Autodesk Inventor part; units mm, degrees
(part 2 of 3)
  line L983 (33.9182, 21.8053) -> (33.8229, 21.957)
  line L984 (33.8229, 21.957) -> (33.7637, 22.1261)
  line L985 (33.7637, 22.1261) -> (33.7437, 22.3041)
  line L986 (33.7437, 22.3041) -> (33.7637, 22.4821)
  line L987 (33.7637, 22.4821) -> (33.8229, 22.6512)
  line L988 (33.8229, 22.6512) -> (33.9182, 22.8029)
  line L989 (33.9182, 22.8029) -> (34.0449, 22.9296)
  line L990 (34.0449, 22.9296) -> (34.1966, 23.0249)
  line L991 (34.1966, 23.0249) -> (34.3656, 23.084)
  line L992 (34.3656, 23.084) -> (34.5437, 23.1041)
  line L993 (34.5437, 23.1041) -> (34.7217, 23.084)
  line L994 (57.188, 32.7799) -> (57.3571, 32.7208)
  line L995 (57.3571, 32.7208) -> (57.5088, 32.6255)
  line L996 (57.5088, 32.6255) -> (57.6355, 32.4988)
  line L997 (57.6355, 32.4988) -> (57.7308, 32.3471)
  line L998 (57.7308, 32.3471) -> (57.7899, 32.178)
  line L999 (57.7899, 32.178) -> (57.81, 32)
  line L1000 (57.81, 32) -> (57.7899, 31.822)
  line L1001 (57.7899, 31.822) -> (57.7308, 31.6529)
  line L1002 (57.7308, 31.6529) -> (57.6355, 31.5012)
  line L1003 (57.6355, 31.5012) -> (57.51, 31.3757)
  line L1004 (57.51, 31.3757) -> (57.51, 30.7979)
  line L1005 (57.51, 30.7979) -> (57.5024, 30.745)
  line L1006 (57.5024, 30.745) -> (57.4986, 30.6916)
  line L1007 (57.4986, 30.6916) -> (57.4923, 30.6748)
  line L1008 (57.4923, 30.6748) -> (57.4897, 30.6571)
  line L1009 (57.4897, 30.6571) -> (57.4675, 30.6084)
  line L1010 (57.4675, 30.6084) -> (57.4488, 30.5583)
  line L1011 (57.4488, 30.5583) -> (57.4381, 30.5439)
  line L1012 (57.4381, 30.5439) -> (57.4306, 30.5276)
  line L1013 (57.4306, 30.5276) -> (57.3956, 30.4872)
  line L1014 (57.3956, 30.4872) -> (57.3636, 30.4444)
  line L1015 (57.3636, 30.4444) -> (52.3656, 25.4464)
  line L1016 (52.3656, 25.4464) -> (52.3228, 25.4144)
  line L1017 (52.3228, 25.4144) -> (52.2824, 25.3794)
  line L1018 (52.2824, 25.3794) -> (52.2661, 25.3719)
  line L1019 (52.2661, 25.3719) -> (52.2517, 25.3612)
  line L1020 (52.2517, 25.3612) -> (52.2016, 25.3425)
  line L1021 (52.2016, 25.3425) -> (52.1529, 25.3203)
  line L1022 (52.1529, 25.3203) -> (52.1352, 25.3177)
  line L1023 (52.1352, 25.3177) -> (52.1184, 25.3114)
  line L1024 (52.1184, 25.3114) -> (52.065, 25.3076)
  line L1025 (52.065, 25.3076) -> (52.0121, 25.3)
  line L1026 (52.0121, 25.3) -> (32.5037, 25.3)
  line L1027 (32.5037, 25.3) -> (32.5037, 22.9283)
  line L1028 (32.5037, 22.9283) -> (32.6291, 22.8029)
  line L1029 (32.6291, 22.8029) -> (32.7244, 22.6512)
  line L1030 (32.7244, 22.6512) -> (32.7836, 22.4821)
  line L1031 (32.7836, 22.4821) -> (32.8037, 22.3041)
  line L1032 (32.8037, 22.3041) -> (32.7836, 22.1261)
  line L1033 (32.7836, 22.1261) -> (32.7244, 21.957)
  line L1034 (32.7244, 21.957) -> (32.6291, 21.8053)
  line L1035 (32.6291, 21.8053) -> (32.5025, 21.6786)
  line L1036 (32.5025, 21.6786) -> (32.3508, 21.5833)
  line L1037 (32.3508, 21.5833) -> (32.1817, 21.5241)
  line L1038 (32.1817, 21.5241) -> (32.0037, 21.5041)
  line L1039 (32.0037, 21.5041) -> (31.8256, 21.5241)
  line L1040 (31.8256, 21.5241) -> (31.6566, 21.5833)
  line L1041 (31.6566, 21.5833) -> (31.5049, 21.6786)
  line L1042 (31.5049, 21.6786) -> (31.3782, 21.8053)
  line L1043 (31.3782, 21.8053) -> (31.2829, 21.957)
  line L1044 (31.2829, 21.957) -> (31.2237, 22.1261)
  line L1045 (31.2237, 22.1261) -> (31.2037, 22.3041)
  line L1046 (31.2037, 22.3041) -> (31.2237, 22.4821)
  line L1047 (31.2237, 22.4821) -> (31.2829, 22.6512)
  line L1048 (31.2829, 22.6512) -> (31.3782, 22.8029)
  line L1049 (31.3782, 22.8029) -> (31.5037, 22.9283)
  line L1050 (31.5037, 22.9283) -> (31.5037, 25.3601)
  line L1051 (31.5037, 25.3601) -> (29.8918, 25.3601)
  line L1052 (29.8918, 25.3601) -> (29.8621, 25.3045)
  line L1053 (29.8621, 25.3045) -> (29.7377, 25.153)
  line L1054 (29.7377, 25.153) -> (29.5862, 25.0286)
  line L1055 (29.5862, 25.0286) -> (29.4133, 24.9362)
  line L1056 (29.4133, 24.9362) -> (29.2257, 24.8793)
  line L1057 (29.2257, 24.8793) -> (29.0306, 24.8601)
  line L1058 (29.0306, 24.8601) -> (28.8355, 24.8793)
  line L1059 (28.8355, 24.8793) -> (28.6479, 24.9362)
  line L1060 (28.6479, 24.9362) -> (28.475, 25.0286)
  line L1061 (28.475, 25.0286) -> (28.3235, 25.153)
  line L1062 (28.3235, 25.153) -> (28.1991, 25.3045)
  line L1063 (28.1991, 25.3045) -> (28.1694, 25.3601)
  line L1064 (28.1694, 25.3601) -> (27.5999, 25.3601)
  line L1065 (27.5999, 25.3601) -> (27.547, 25.3677)
  line L1066 (27.547, 25.3677) -> (27.4936, 25.3715)
  line L1067 (27.4936, 25.3715) -> (27.4768, 25.3778)
  line L1068 (27.4768, 25.3778) -> (27.459, 25.3803)
  line L1069 (27.459, 25.3803) -> (27.4104, 25.4026)
  line L1070 (27.4104, 25.4026) -> (27.3603, 25.4213)
  line L1071 (27.3603, 25.4213) -> (27.3459, 25.432)
  line L1072 (27.3459, 25.432) -> (27.3296, 25.4395)
  line L1073 (27.3296, 25.4395) -> (27.2892, 25.4745)
  line L1074 (27.2892, 25.4745) -> (27.2464, 25.5065)
  line L1075 (27.2464, 25.5065) -> (21.5935, 31.1594)
  line L1076 (21.5935, 31.1594) -> (21.51, 31.15)
  line L1077 (21.51, 31.15) -> (21.332, 31.1701)
  line L1078 (21.332, 31.1701) -> (21.1629, 31.2292)
  line L1079 (21.1629, 31.2292) -> (21.0112, 31.3245)
  line L1080 (21.0112, 31.3245) -> (20.8857, 31.45)
  line L1081 (20.8857, 31.45) -> (20.7171, 31.45)
  line L1082 (20.7171, 31.45) -> (15.5506, 26.2835)
  line L1083 (15.5506, 26.2835) -> (15.56, 26.2)
  line L1084 (15.56, 26.2) -> (15.5399, 26.022)
  line L1085 (15.5399, 26.022) -> (15.4808, 25.8529)
  line L1086 (15.4808, 25.8529) -> (15.3855, 25.7012)
  line L1087 (15.3855, 25.7012) -> (15.2588, 25.5745)
  line L1088 (15.2588, 25.5745) -> (15.1071, 25.4792)
  line L1089 (15.1071, 25.4792) -> (14.938, 25.4201)
  line L1090 (14.938, 25.4201) -> (14.76, 25.4)
  line L1091 (14.76, 25.4) -> (14.582, 25.4201)
  line L1092 (14.582, 25.4201) -> (14.4129, 25.4792)
  line L1093 (14.4129, 25.4792) -> (14.2612, 25.5745)
  line L1094 (14.2612, 25.5745) -> (14.1345, 25.7012)
  line L1095 (14.1345, 25.7012) -> (14.0392, 25.8529)
  line L1096 (14.0392, 25.8529) -> (13.9801, 26.022)
  line L1097 (13.9801, 26.022) -> (13.96, 26.2)
  line L1098 (13.96, 26.2) -> (13.9801, 26.378)
  line L1099 (13.9801, 26.378) -> (14.0392, 26.5471)
  line L1100 (14.0392, 26.5471) -> (14.1345, 26.6988)
  line L1101 (14.1345, 26.6988) -> (14.2612, 26.8255)
  line L1102 (14.2612, 26.8255) -> (14.4129, 26.9208)
  line L1103 (14.4129, 26.9208) -> (14.582, 26.9799)
  line L1104 (14.582, 26.9799) -> (14.76, 27)
  line L1105 (14.76, 27) -> (14.8435, 26.9906)
  line L1106 (14.8435, 26.9906) -> (20.1564, 32.3036)
  line L1107 (20.1564, 32.3036) -> (20.1993, 32.3356)
  line L1108 (20.1993, 32.3356) -> (20.2397, 32.3706)
  line L1109 (20.2397, 32.3706) -> (20.256, 32.3781)
  line L1110 (20.256, 32.3781) -> (20.2704, 32.3888)
  line L1111 (20.2704, 32.3888) -> (20.3205, 32.4075)
  line L1112 (20.3205, 32.4075) -> (20.3691, 32.4297)
  line L1113 (20.3691, 32.4297) -> (20.3869, 32.4323)
  line L1114 (20.3869, 32.4323) -> (20.4037, 32.4386)
  line L1115 (20.4037, 32.4386) -> (20.4571, 32.4424)
  line L1116 (20.4571, 32.4424) -> (20.51, 32.45)
  line L1117 (20.51, 32.45) -> (20.8857, 32.45)
  line L1118 (20.8857, 32.45) -> (21.0112, 32.5755)
  line L1119 (21.0112, 32.5755) -> (21.1629, 32.6708)
  line L1120 (21.1629, 32.6708) -> (21.332, 32.7299)
  line L1121 (21.332, 32.7299) -> (21.51, 32.75)
  line L1122 (21.51, 32.75) -> (21.688, 32.7299)
  line L1123 (21.688, 32.7299) -> (21.8571, 32.6708)
  line L1124 (21.8571, 32.6708) -> (22.0088, 32.5755)
  line L1125 (22.0088, 32.5755) -> (22.1355, 32.4488)
  line L1126 (22.1355, 32.4488) -> (22.2308, 32.2971)
  line L1127 (22.2308, 32.2971) -> (22.2899, 32.128)
  line L1128 (22.2899, 32.128) -> (22.31, 31.95)
  line L1129 (22.31, 31.95) -> (22.3006, 31.8665)
  line L1130 (22.3006, 31.8665) -> (27.807, 26.3601)
  line L1131 (27.807, 26.3601) -> (28.1694, 26.3601)
  line L1132 (28.1694, 26.3601) -> (28.1991, 26.4157)
  line L1133 (28.1991, 26.4157) -> (28.3235, 26.5672)
  line L1134 (28.3235, 26.5672) -> (28.475, 26.6916)
  line L1135 (28.475, 26.6916) -> (28.6479, 26.784)
  line L1136 (28.6479, 26.784) -> (28.8355, 26.8409)
  line L1137 (28.8355, 26.8409) -> (29.0306, 26.8601)
  line L1138 (29.0306, 26.8601) -> (29.2257, 26.8409)
  line L1139 (29.2257, 26.8409) -> (29.4133, 26.784)
  line L1140 (29.4133, 26.784) -> (29.5862, 26.6916)
  line L1141 (29.5862, 26.6916) -> (29.7377, 26.5672)
  line L1142 (29.7377, 26.5672) -> (29.8621, 26.4157)
  line L1143 (29.8621, 26.4157) -> (29.8918, 26.3601)
  line L1144 (29.8918, 26.3601) -> (31.8972, 26.3601)
  line L1145 (31.8972, 26.3601) -> (31.9502, 26.3525)
  line L1146 (31.9502, 26.3525) -> (32.0035, 26.3487)
  line L1147 (32.0035, 26.3487) -> (32.0203, 26.3424)
  line L1148 (32.0203, 26.3424) -> (32.0381, 26.3398)
  line L1149 (32.0381, 26.3398) -> (32.0867, 26.3176)
  line L1150 (32.0867, 26.3176) -> (32.134, 26.3)
  line L1151 (32.134, 26.3) -> (51.805, 26.3)
  line L1152 (51.805, 26.3) -> (56.51, 31.005)
  line L1153 (56.51, 31.005) -> (56.51, 31.3757)
  line L1154 (56.51, 31.3757) -> (56.3845, 31.5012)
  line L1155 (56.3845, 31.5012) -> (56.2892, 31.6529)
  line L1156 (56.2892, 31.6529) -> (56.2301, 31.822)
  line L1157 (56.2301, 31.822) -> (56.21, 32)
  line L1158 (56.21, 32) -> (56.2301, 32.178)
  line L1159 (56.2301, 32.178) -> (56.2892, 32.3471)
  line L1160 (56.2892, 32.3471) -> (56.3845, 32.4988)
  line L1161 (56.3845, 32.4988) -> (56.5112, 32.6255)
  line L1162 (56.5112, 32.6255) -> (56.6629, 32.7208)
  line L1163 (56.6629, 32.7208) -> (56.832, 32.7799)
  line L1164 (56.832, 32.7799) -> (57.01, 32.8)
  line L1165 (57.01, 32.8) -> (57.188, 32.7799)
  line L1166 (29.6417, 23.084) -> (29.8108, 23.0249)
  line L1167 (29.8108, 23.0249) -> (29.9625, 22.9296)
  line L1168 (29.9625, 22.9296) -> (30.0891, 22.8029)
  line L1169 (30.0891, 22.8029) -> (30.1844, 22.6512)
  line L1170 (30.1844, 22.6512) -> (30.2436, 22.4821)
  line L1171 (30.2436, 22.4821) -> (30.2637, 22.3041)
  line L1172 (30.2637, 22.3041) -> (30.2436, 22.1261)
  line L1173 (30.2436, 22.1261) -> (30.1844, 21.957)
  line L1174 (30.1844, 21.957) -> (30.0891, 21.8053)
  line L1175 (30.0891, 21.8053) -> (29.9625, 21.6786)
  line L1176 (29.9625, 21.6786) -> (29.8108, 21.5833)
  line L1177 (29.8108, 21.5833) -> (29.6417, 21.5241)
  line L1178 (29.6417, 21.5241) -> (29.4637, 21.5041)
  line L1179 (29.4637, 21.5041) -> (29.2856, 21.5241)
  line L1180 (29.2856, 21.5241) -> (29.1166, 21.5833)
  line L1181 (29.1166, 21.5833) -> (28.9649, 21.6786)
  line L1182 (28.9649, 21.6786) -> (28.8382, 21.8053)
  line L1183 (28.8382, 21.8053) -> (28.7429, 21.957)
  line L1184 (28.7429, 21.957) -> (28.6837, 22.1261)
  line L1185 (28.6837, 22.1261) -> (28.6637, 22.3041)
  line L1186 (28.6637, 22.3041) -> (28.6837, 22.4821)
  line L1187 (28.6837, 22.4821) -> (28.7429, 22.6512)
  line L1188 (28.7429, 22.6512) -> (28.8382, 22.8029)
  line L1189 (28.8382, 22.8029) -> (28.9649, 22.9296)
  line L1190 (28.9649, 22.9296) -> (29.1166, 23.0249)
  line L1191 (29.1166, 23.0249) -> (29.2856, 23.084)
  line L1192 (29.2856, 23.084) -> (29.4637, 23.1041)
  line L1193 (29.4637, 23.1041) -> (29.6417, 23.084)
  line L1194 (27.1017, 23.084) -> (27.2708, 23.0249)
  line L1195 (27.2708, 23.0249) -> (27.4225, 22.9296)
  line L1196 (27.4225, 22.9296) -> (27.5491, 22.8029)
  line L1197 (27.5491, 22.8029) -> (27.6444, 22.6512)
  line L1198 (27.6444, 22.6512) -> (27.7036, 22.4821)
  line L1199 (27.7036, 22.4821) -> (27.7237, 22.3041)
  line L1200 (27.7237, 22.3041) -> (27.7036, 22.1261)
  line L1201 (27.7036, 22.1261) -> (27.6444, 21.957)
  line L1202 (27.6444, 21.957) -> (27.5491, 21.8053)
  line L1203 (27.5491, 21.8053) -> (27.4225, 21.6786)
  line L1204 (27.4225, 21.6786) -> (27.2708, 21.5833)
  line L1205 (27.2708, 21.5833) -> (27.1017, 21.5241)
  line L1206 (27.1017, 21.5241) -> (26.9237, 21.5041)
  line L1207 (26.9237, 21.5041) -> (26.7456, 21.5241)
  line L1208 (26.7456, 21.5241) -> (26.5766, 21.5833)
  line L1209 (26.5766, 21.5833) -> (26.4249, 21.6786)
  line L1210 (26.4249, 21.6786) -> (26.2982, 21.8053)
  line L1211 (26.2982, 21.8053) -> (26.2029, 21.957)
  line L1212 (26.2029, 21.957) -> (26.1437, 22.1261)
  line L1213 (26.1437, 22.1261) -> (26.1237, 22.3041)
  line L1214 (26.1237, 22.3041) -> (26.1437, 22.4821)
  line L1215 (26.1437, 22.4821) -> (26.2029, 22.6512)
  line L1216 (26.2029, 22.6512) -> (26.2982, 22.8029)
  line L1217 (26.2982, 22.8029) -> (26.4249, 22.9296)
  line L1218 (26.4249, 22.9296) -> (26.5766, 23.0249)
  line L1219 (26.5766, 23.0249) -> (26.7456, 23.084)
  line L1220 (26.7456, 23.084) -> (26.9237, 23.1041)
  line L1221 (26.9237, 23.1041) -> (27.1017, 23.084)
  line L1222 (24.5617, 23.084) -> (24.7308, 23.0249)
  line L1223 (24.7308, 23.0249) -> (24.8825, 22.9296)
  line L1224 (24.8825, 22.9296) -> (25.0091, 22.8029)
  line L1225 (25.0091, 22.8029) -> (25.1044, 22.6512)
  line L1226 (25.1044, 22.6512) -> (25.1636, 22.4821)
  line L1227 (25.1636, 22.4821) -> (25.1837, 22.3041)
  line L1228 (25.1837, 22.3041) -> (25.1636, 22.1261)
  line L1229 (25.1636, 22.1261) -> (25.1044, 21.957)
  line L1230 (25.1044, 21.957) -> (25.0091, 21.8053)
  line L1231 (25.0091, 21.8053) -> (24.8825, 21.6786)
  line L1232 (24.8825, 21.6786) -> (24.7308, 21.5833)
  line L1233 (24.7308, 21.5833) -> (24.5617, 21.5241)
  line L1234 (24.5617, 21.5241) -> (24.3837, 21.5041)
  line L1235 (24.3837, 21.5041) -> (24.2056, 21.5241)
  line L1236 (24.2056, 21.5241) -> (24.0366, 21.5833)
  line L1237 (24.0366, 21.5833) -> (23.8849, 21.6786)
  line L1238 (23.8849, 21.6786) -> (23.7582, 21.8053)
  line L1239 (23.7582, 21.8053) -> (23.6629, 21.957)
  line L1240 (23.6629, 21.957) -> (23.6037, 22.1261)
  line L1241 (23.6037, 22.1261) -> (23.5837, 22.3041)
  line L1242 (23.5837, 22.3041) -> (23.6037, 22.4821)
  line L1243 (23.6037, 22.4821) -> (23.6629, 22.6512)
  line L1244 (23.6629, 22.6512) -> (23.7582, 22.8029)
  line L1245 (23.7582, 22.8029) -> (23.8849, 22.9296)
  line L1246 (23.8849, 22.9296) -> (24.0366, 23.0249)
  line L1247 (24.0366, 23.0249) -> (24.2056, 23.084)
  line L1248 (24.2056, 23.084) -> (24.3837, 23.1041)
  line L1249 (24.3837, 23.1041) -> (24.5617, 23.084)
  line L1250 (22.0217, 23.084) -> (22.1908, 23.0249)
  line L1251 (22.1908, 23.0249) -> (22.3425, 22.9296)
  line L1252 (22.3425, 22.9296) -> (22.4691, 22.8029)
  line L1253 (22.4691, 22.8029) -> (22.5644, 22.6512)
  line L1254 (22.5644, 22.6512) -> (22.6236, 22.4821)
  line L1255 (22.6236, 22.4821) -> (22.6437, 22.3041)
  line L1256 (22.6437, 22.3041) -> (22.6236, 22.1261)
  line L1257 (22.6236, 22.1261) -> (22.5644, 21.957)
  line L1258 (22.5644, 21.957) -> (22.4691, 21.8053)
  line L1259 (22.4691, 21.8053) -> (22.3425, 21.6786)
  line L1260 (22.3425, 21.6786) -> (22.1908, 21.5833)
  line L1261 (22.1908, 21.5833) -> (22.0217, 21.5241)
  line L1262 (22.0217, 21.5241) -> (21.8437, 21.5041)
  line L1263 (21.8437, 21.5041) -> (21.6656, 21.5241)
  line L1264 (21.6656, 21.5241) -> (21.4966, 21.5833)
  line L1265 (21.4966, 21.5833) -> (21.3449, 21.6786)
  line L1266 (21.3449, 21.6786) -> (21.2182, 21.8053)
  line L1267 (21.2182, 21.8053) -> (21.1229, 21.957)
  line L1268 (21.1229, 21.957) -> (21.0637, 22.1261)
  line L1269 (21.0637, 22.1261) -> (21.0437, 22.3041)
  line L1270 (21.0437, 22.3041) -> (21.0637, 22.4821)
  line L1271 (21.0637, 22.4821) -> (21.1229, 22.6512)
  line L1272 (21.1229, 22.6512) -> (21.2182, 22.8029)
  line L1273 (21.2182, 22.8029) -> (21.3449, 22.9296)
  line L1274 (21.3449, 22.9296) -> (21.4966, 23.0249)
  line L1275 (21.4966, 23.0249) -> (21.6656, 23.084)
  line L1276 (21.6656, 23.084) -> (21.8437, 23.1041)
  line L1277 (21.8437, 23.1041) -> (22.0217, 23.084)
  line L1278 (19.4817, 23.084) -> (19.6508, 23.0249)
  line L1279 (19.6508, 23.0249) -> (19.8025, 22.9296)
  line L1280 (19.8025, 22.9296) -> (19.9291, 22.8029)
  line L1281 (19.9291, 22.8029) -> (20.0244, 22.6512)
  line L1282 (20.0244, 22.6512) -> (20.0836, 22.4821)
  line L1283 (20.0836, 22.4821) -> (20.1037, 22.3041)
  line L1284 (20.1037, 22.3041) -> (20.0836, 22.1261)
  line L1285 (20.0836, 22.1261) -> (20.0244, 21.957)
  line L1286 (20.0244, 21.957) -> (19.9291, 21.8053)
  line L1287 (19.9291, 21.8053) -> (19.8025, 21.6786)
  line L1288 (19.8025, 21.6786) -> (19.6508, 21.5833)
  line L1289 (19.6508, 21.5833) -> (19.4817, 21.5241)
  line L1290 (19.4817, 21.5241) -> (19.3037, 21.5041)
  line L1291 (19.3037, 21.5041) -> (19.1256, 21.5241)
  line L1292 (19.1256, 21.5241) -> (18.9566, 21.5833)
  line L1293 (18.9566, 21.5833) -> (18.8049, 21.6786)
  line L1294 (18.8049, 21.6786) -> (18.6782, 21.8053)
  line L1295 (18.6782, 21.8053) -> (18.5829, 21.957)
  line L1296 (18.5829, 21.957) -> (18.5237, 22.1261)
  line L1297 (18.5237, 22.1261) -> (18.5037, 22.3041)
  line L1298 (18.5037, 22.3041) -> (18.5237, 22.4821)
  line L1299 (18.5237, 22.4821) -> (18.5829, 22.6512)
  line L1300 (18.5829, 22.6512) -> (18.6782, 22.8029)
  line L1301 (18.6782, 22.8029) -> (18.8049, 22.9296)
  line L1302 (18.8049, 22.9296) -> (18.9566, 23.0249)
  line L1303 (18.9566, 23.0249) -> (19.1256, 23.084)
  line L1304 (19.1256, 23.084) -> (19.3037, 23.1041)
  line L1305 (19.3037, 23.1041) -> (19.4817, 23.084)
  line L1306 (22.4306, 24.8601) -> (20.4306, 24.8601)
  line L1307 (20.4306, 24.8601) -> (20.4306, 25.2639)
  line L1308 (20.4306, 25.2639) -> (17.5543, 22.3876)
  line L1309 (17.5543, 22.3876) -> (17.5637, 22.3041)
  line L1310 (17.5637, 22.3041) -> (17.5436, 22.1261)
  line L1311 (17.5436, 22.1261) -> (17.4844, 21.957)
  line L1312 (17.4844, 21.957) -> (17.3891, 21.8053)
  line L1313 (17.3891, 21.8053) -> (17.2625, 21.6786)
  line L1314 (17.2625, 21.6786) -> (17.1108, 21.5833)
  line L1315 (17.1108, 21.5833) -> (16.9417, 21.5241)
  line L1316 (16.9417, 21.5241) -> (16.7637, 21.5041)
  line L1317 (16.7637, 21.5041) -> (16.5856, 21.5241)
  line L1318 (16.5856, 21.5241) -> (16.4166, 21.5833)
  line L1319 (16.4166, 21.5833) -> (16.2649, 21.6786)
  line L1320 (16.2649, 21.6786) -> (16.1382, 21.8053)
  line L1321 (16.1382, 21.8053) -> (16.0429, 21.957)
  line L1322 (16.0429, 21.957) -> (15.9837, 22.1261)
  line L1323 (15.9837, 22.1261) -> (15.9637, 22.3041)
  line L1324 (15.9637, 22.3041) -> (15.9837, 22.4821)
  line L1325 (15.9837, 22.4821) -> (16.0429, 22.6512)
  line L1326 (16.0429, 22.6512) -> (16.1382, 22.8029)
  line L1327 (16.1382, 22.8029) -> (16.2649, 22.9296)
  line L1328 (16.2649, 22.9296) -> (16.4166, 23.0249)
  line L1329 (16.4166, 23.0249) -> (16.5856, 23.084)
  line L1330 (16.5856, 23.084) -> (16.7637, 23.1041)
  line L1331 (16.7637, 23.1041) -> (16.8471, 23.0947)
  line L1332 (16.8471, 23.0947) -> (19.9661, 26.2136)
  line L1333 (19.9661, 26.2136) -> (20.0089, 26.2457)
  line L1334 (20.0089, 26.2457) -> (20.0493, 26.2807)
  line L1335 (20.0493, 26.2807) -> (20.0657, 26.2882)
  line L1336 (20.0657, 26.2882) -> (20.08, 26.2989)
  line L1337 (20.08, 26.2989) -> (20.1301, 26.3176)
  line L1338 (20.1301, 26.3176) -> (20.1788, 26.3398)
  line L1339 (20.1788, 26.3398) -> (20.1966, 26.3424)
  line L1340 (20.1966, 26.3424) -> (20.2134, 26.3487)
  line L1341 (20.2134, 26.3487) -> (20.2667, 26.3525)
  line L1342 (20.2667, 26.3525) -> (20.3197, 26.3601)
  line L1343 (20.3197, 26.3601) -> (20.4306, 26.3601)
  line L1344 (20.4306, 26.3601) -> (20.4306, 26.8601)
  line L1345 (20.4306, 26.8601) -> (22.4306, 26.8601)
  line L1346 (22.4306, 26.8601) -> (22.4306, 24.8601)
  line L1347 (21.068, 29.3799) -> (21.2371, 29.3208)
  line L1348 (21.2371, 29.3208) -> (21.3888, 29.2255)
  line L1349 (21.3888, 29.2255) -> (21.5155, 29.0988)
  line L1350 (21.5155, 29.0988) -> (21.6108, 28.9471)
  line L1351 (21.6108, 28.9471) -> (21.6699, 28.778)
  line L1352 (21.6699, 28.778) -> (21.69, 28.6)
  line L1353 (21.69, 28.6) -> (21.6699, 28.422)
  line L1354 (21.6699, 28.422) -> (21.6108, 28.2529)
  line L1355 (21.6108, 28.2529) -> (21.5155, 28.1012)
  line L1356 (21.5155, 28.1012) -> (21.3888, 27.9745)
  line L1357 (21.3888, 27.9745) -> (21.2371, 27.8792)
  line L1358 (21.2371, 27.8792) -> (21.068, 27.8201)
  line L1359 (21.068, 27.8201) -> (20.89, 27.8)
  line L1360 (20.89, 27.8) -> (20.712, 27.8201)
  line L1361 (20.712, 27.8201) -> (20.5429, 27.8792)
  line L1362 (20.5429, 27.8792) -> (20.5202, 27.8935)
  line L1363 (20.5202, 27.8935) -> (15.0143, 22.3876)
  line L1364 (15.0143, 22.3876) -> (15.0237, 22.3041)
  line L1365 (15.0237, 22.3041) -> (15.0036, 22.1261)
  line L1366 (15.0036, 22.1261) -> (14.9444, 21.957)
  line L1367 (14.9444, 21.957) -> (14.8491, 21.8053)
  line L1368 (14.8491, 21.8053) -> (14.7225, 21.6786)
  line L1369 (14.7225, 21.6786) -> (14.5708, 21.5833)
  line L1370 (14.5708, 21.5833) -> (14.4017, 21.5241)
  line L1371 (14.4017, 21.5241) -> (14.2237, 21.5041)
  line L1372 (14.2237, 21.5041) -> (14.0456, 21.5241)
  line L1373 (14.0456, 21.5241) -> (13.8766, 21.5833)
  line L1374 (13.8766, 21.5833) -> (13.7249, 21.6786)
  line L1375 (13.7249, 21.6786) -> (13.5982, 21.8053)
  line L1376 (13.5982, 21.8053) -> (13.5029, 21.957)
  line L1377 (13.5029, 21.957) -> (13.4437, 22.1261)
  line L1378 (13.4437, 22.1261) -> (13.4237, 22.3041)
  line L1379 (13.4237, 22.3041) -> (13.4437, 22.4821)
  line L1380 (13.4437, 22.4821) -> (13.5029, 22.6512)
  line L1381 (13.5029, 22.6512) -> (13.5982, 22.8029)
  line L1382 (13.5982, 22.8029) -> (13.7249, 22.9296)
  line L1383 (13.7249, 22.9296) -> (13.8766, 23.0249)
  line L1384 (13.8766, 23.0249) -> (14.0456, 23.084)
  line L1385 (14.0456, 23.084) -> (14.2237, 23.1041)
  line L1386 (14.2237, 23.1041) -> (14.3071, 23.0947)
  line L1387 (14.3071, 23.0947) -> (20.166, 28.9536)
  line L1388 (20.166, 28.9536) -> (20.1797, 28.9638)
  line L1389 (20.1797, 28.9638) -> (20.2645, 29.0988)
  line L1390 (20.2645, 29.0988) -> (20.3912, 29.2255)
  line L1391 (20.3912, 29.2255) -> (20.5429, 29.3208)
  line L1392 (20.5429, 29.3208) -> (20.712, 29.3799)
  line L1393 (20.712, 29.3799) -> (20.89, 29.4)
  line L1394 (20.89, 29.4) -> (21.068, 29.3799)
  line L1395 (14.068, 32.7299) -> (14.2371, 32.6708)
  line L1396 (14.2371, 32.6708) -> (14.3888, 32.5755)
  line L1397 (14.3888, 32.5755) -> (14.5155, 32.4488)
  line L1398 (14.5155, 32.4488) -> (14.6108, 32.2971)
  line L1399 (14.6108, 32.2971) -> (14.6699, 32.128)
  line L1400 (14.6699, 32.128) -> (14.69, 31.95)
  line L1401 (14.69, 31.95) -> (14.6699, 31.772)
  line L1402 (14.6699, 31.772) -> (14.6108, 31.6029)
  line L1403 (14.6108, 31.6029) -> (14.5155, 31.4512)
  line L1404 (14.5155, 31.4512) -> (14.3888, 31.3245)
  line L1405 (14.3888, 31.3245) -> (14.2371, 31.2292)
  line L1406 (14.2371, 31.2292) -> (14.068, 31.1701)
  line L1407 (14.068, 31.1701) -> (13.89, 31.15)
  line L1408 (13.89, 31.15) -> (13.712, 31.1701)
  line L1409 (13.712, 31.1701) -> (13.5429, 31.2292)
  line L1410 (13.5429, 31.2292) -> (13.3912, 31.3245)
  line L1411 (13.3912, 31.3245) -> (13.3199, 31.3959)
  line L1412 (13.3199, 31.3959) -> (11.4316, 29.5076)
  line L1413 (11.4316, 29.5076) -> (11.441, 29.4241)
  line L1414 (11.441, 29.4241) -> (11.4209, 29.2461)
  line L1415 (11.4209, 29.2461) -> (11.3617, 29.077)
  line L1416 (11.3617, 29.077) -> (11.2664, 28.9253)
  line L1417 (11.2664, 28.9253) -> (11.141, 28.7998)
  line L1418 (11.141, 28.7998) -> (11.141, 26.9661)
  line L1419 (11.141, 26.9661) -> (12.0372, 26.0699)
  line L1420 (12.0372, 26.0699) -> (12.0693, 26.0271)
  line L1421 (12.0693, 26.0271) -> (12.1043, 25.9867)
  line L1422 (12.1043, 25.9867) -> (12.1117, 25.9703)
  line L1423 (12.1117, 25.9703) -> (12.1225, 25.956)
  line L1424 (12.1225, 25.956) -> (12.1412, 25.9059)
  line L1425 (12.1412, 25.9059) -> (12.1634, 25.8572)
  line L1426 (12.1634, 25.8572) -> (12.166, 25.8394)
  line L1427 (12.166, 25.8394) -> (12.1722, 25.8226)
  line L1428 (12.1722, 25.8226) -> (12.176, 25.7693)
  line L1429 (12.176, 25.7693) -> (12.1837, 25.7163)
  line L1430 (12.1837, 25.7163) -> (12.1837, 22.9283)
  line L1431 (12.1837, 22.9283) -> (12.3091, 22.8029)
  line L1432 (12.3091, 22.8029) -> (12.4044, 22.6512)
  line L1433 (12.4044, 22.6512) -> (12.4636, 22.4821)
  line L1434 (12.4636, 22.4821) -> (12.4837, 22.3041)
  line L1435 (12.4837, 22.3041) -> (12.4636, 22.1261)
  line L1436 (12.4636, 22.1261) -> (12.4044, 21.957)
  line L1437 (12.4044, 21.957) -> (12.3091, 21.8053)
  line L1438 (12.3091, 21.8053) -> (12.1825, 21.6786)
  line L1439 (12.1825, 21.6786) -> (12.0308, 21.5833)
  line L1440 (12.0308, 21.5833) -> (11.8617, 21.5241)
  line L1441 (11.8617, 21.5241) -> (11.6837, 21.5041)
  line L1442 (11.6837, 21.5041) -> (11.5056, 21.5241)
  line L1443 (11.5056, 21.5241) -> (11.3366, 21.5833)
  line L1444 (11.3366, 21.5833) -> (11.1849, 21.6786)
  line L1445 (11.1849, 21.6786) -> (11.0582, 21.8053)
  line L1446 (11.0582, 21.8053) -> (10.9629, 21.957)
  line L1447 (10.9629, 21.957) -> (10.9037, 22.1261)
  line L1448 (10.9037, 22.1261) -> (10.8837, 22.3041)
  line L1449 (10.8837, 22.3041) -> (10.9037, 22.4821)
  line L1450 (10.9037, 22.4821) -> (10.9629, 22.6512)
  line L1451 (10.9629, 22.6512) -> (11.0582, 22.8029)
  line L1452 (11.0582, 22.8029) -> (11.1837, 22.9283)
  line L1453 (11.1837, 22.9283) -> (11.1837, 25.5092)
  line L1454 (11.1837, 25.5092) -> (10.2874, 26.4055)
  line L1455 (10.2874, 26.4055) -> (10.2554, 26.4483)
  line L1456 (10.2554, 26.4483) -> (10.2203, 26.4887)
  line L1457 (10.2203, 26.4887) -> (10.2129, 26.505)
  line L1458 (10.2129, 26.505) -> (10.2021, 26.5194)
  line L1459 (10.2021, 26.5194) -> (10.1834, 26.5695)
  line L1460 (10.1834, 26.5695) -> (10.1612, 26.6182)
  line L1461 (10.1612, 26.6182) -> (10.1587, 26.6359)
  line L1462 (10.1587, 26.6359) -> (10.1524, 26.6528)
  line L1463 (10.1524, 26.6528) -> (10.1486, 26.7061)
  line L1464 (10.1486, 26.7061) -> (10.141, 26.759)
  line L1465 (10.141, 26.759) -> (10.141, 28.7998)
  line L1466 (10.141, 28.7998) -> (10.0155, 28.9253)
  line L1467 (10.0155, 28.9253) -> (9.9202, 29.077)
  line L1468 (9.9202, 29.077) -> (9.861, 29.2461)
  line L1469 (9.861, 29.2461) -> (9.841, 29.4241)
  line L1470 (9.841, 29.4241) -> (9.861, 29.6021)
  line L1471 (9.861, 29.6021) -> (9.9202, 29.7712)
  line L1472 (9.9202, 29.7712) -> (10.0155, 29.9229)
  line L1473 (10.0155, 29.9229) -> (10.1422, 30.0496)
  line L1474 (10.1422, 30.0496) -> (10.2939, 30.1449)
  line L1475 (10.2939, 30.1449) -> (10.4629, 30.204)
  line L1476 (10.4629, 30.204) -> (10.641, 30.2241)
  line L1477 (10.641, 30.2241) -> (10.7244, 30.2147)
  line L1478 (10.7244, 30.2147) -> (12.8133, 32.3036)
  line L1479 (12.8133, 32.3036) -> (12.8561, 32.3356)
  line L1480 (12.8561, 32.3356) -> (12.8965, 32.3706)
  line L1481 (12.8965, 32.3706) -> (12.9129, 32.3781)
  line L1482 (12.9129, 32.3781) -> (12.9272, 32.3888)
  line L1483 (12.9272, 32.3888) -> (12.9774, 32.4075)
  line L1484 (12.9774, 32.4075) -> (13.026, 32.4297)
  line L1485 (13.026, 32.4297) -> (13.0438, 32.4323)
  line L1486 (13.0438, 32.4323) -> (13.0606, 32.4386)
  line L1487 (13.0606, 32.4386) -> (13.1139, 32.4424)
  line L1488 (13.1139, 32.4424) -> (13.1669, 32.45)
  line L1489 (13.1669, 32.45) -> (13.2657, 32.45)
  line L1490 (13.2657, 32.45) -> (13.3912, 32.5755)
  line L1491 (13.3912, 32.5755) -> (13.5429, 32.6708)
  line L1492 (13.5429, 32.6708) -> (13.712, 32.7299)
  line L1493 (13.712, 32.7299) -> (13.89, 32.75)
  line L1494 (13.89, 32.75) -> (14.068, 32.7299)
  line L1495 (6.411, 28.5741) -> (6.061, 28.5741)
  line L1496 (6.061, 28.5741) -> (6.061, 27.9861)
  line L1497 (6.061, 27.9861) -> (7.0565, 26.9906)
  line L1498 (7.0565, 26.9906) -> (7.14, 27)
  line L1499 (7.14, 27) -> (7.318, 26.9799)
  line L1500 (7.318, 26.9799) -> (7.4871, 26.9208)
  line L1501 (7.4871, 26.9208) -> (7.6388, 26.8255)
  line L1502 (7.6388, 26.8255) -> (7.7655, 26.6988)
  line L1503 (7.7655, 26.6988) -> (7.8608, 26.5471)
  line L1504 (7.8608, 26.5471) -> (7.9199, 26.378)
  line L1505 (7.9199, 26.378) -> (7.94, 26.2)
  line L1506 (7.94, 26.2) -> (7.9306, 26.1165)
  line L1507 (7.9306, 26.1165) -> (9.4972, 24.5499)
  line L1508 (9.4972, 24.5499) -> (9.5293, 24.5071)
  line L1509 (9.5293, 24.5071) -> (9.5643, 24.4667)
  line L1510 (9.5643, 24.4667) -> (9.5717, 24.4503)
  line L1511 (9.5717, 24.4503) -> (9.5825, 24.436)
  line L1512 (9.5825, 24.436) -> (9.6012, 24.3859)
  line L1513 (9.6012, 24.3859) -> (9.6234, 24.3372)
  line L1514 (9.6234, 24.3372) -> (9.626, 24.3194)
  line L1515 (9.626, 24.3194) -> (9.6322, 24.3026)
  line L1516 (9.6322, 24.3026) -> (9.636, 24.2493)
  line L1517 (9.636, 24.2493) -> (9.6437, 24.1963)
  line L1518 (9.6437, 24.1963) -> (9.6437, 22.9283)
  line L1519 (9.6437, 22.9283) -> (9.7691, 22.8029)
  line L1520 (9.7691, 22.8029) -> (9.8644, 22.6512)
  line L1521 (9.8644, 22.6512) -> (9.9236, 22.4821)
  line L1522 (9.9236, 22.4821) -> (9.9437, 22.3041)
  line L1523 (9.9437, 22.3041) -> (9.9236, 22.1261)
  line L1524 (9.9236, 22.1261) -> (9.8644, 21.957)
  line L1525 (9.8644, 21.957) -> (9.7691, 21.8053)
  line L1526 (9.7691, 21.8053) -> (9.6425, 21.6786)
  line L1527 (9.6425, 21.6786) -> (9.4908, 21.5833)
  line L1528 (9.4908, 21.5833) -> (9.3217, 21.5241)
  line L1529 (9.3217, 21.5241) -> (9.1437, 21.5041)
  line L1530 (9.1437, 21.5041) -> (8.9656, 21.5241)
  line L1531 (8.9656, 21.5241) -> (8.7965, 21.5833)
  line L1532 (8.7965, 21.5833) -> (8.6449, 21.6786)
  line L1533 (8.6449, 21.6786) -> (8.5182, 21.8053)
  line L1534 (8.5182, 21.8053) -> (8.4229, 21.957)
  line L1535 (8.4229, 21.957) -> (8.3637, 22.1261)
  line L1536 (8.3637, 22.1261) -> (8.3437, 22.3041)
  line L1537 (8.3437, 22.3041) -> (8.3637, 22.4821)
  line L1538 (8.3637, 22.4821) -> (8.4229, 22.6512)
  line L1539 (8.4229, 22.6512) -> (8.5182, 22.8029)
  line L1540 (8.5182, 22.8029) -> (8.6437, 22.9283)
  line L1541 (8.6437, 22.9283) -> (8.6437, 23.9892)
  line L1542 (8.6437, 23.9892) -> (7.2235, 25.4094)
  line L1543 (7.2235, 25.4094) -> (7.14, 25.4)
  line L1544 (7.14, 25.4) -> (6.962, 25.4201)
  line L1545 (6.962, 25.4201) -> (6.7929, 25.4792)
  line L1546 (6.7929, 25.4792) -> (6.6412, 25.5745)
  line L1547 (6.6412, 25.5745) -> (6.5145, 25.7012)
  line L1548 (6.5145, 25.7012) -> (6.4192, 25.8529)
  line L1549 (6.4192, 25.8529) -> (6.3601, 26.022)
  line L1550 (6.3601, 26.022) -> (6.34, 26.2)
  line L1551 (6.34, 26.2) -> (6.3494, 26.2835)
  line L1552 (6.3494, 26.2835) -> (5.2074, 27.4255)
  line L1553 (5.2074, 27.4255) -> (5.1754, 27.4683)
  line L1554 (5.1754, 27.4683) -> (5.1403, 27.5087)
  line L1555 (5.1403, 27.5087) -> (5.1329, 27.5251)
  line L1556 (5.1329, 27.5251) -> (5.1221, 27.5394)
  line L1557 (5.1221, 27.5394) -> (5.1034, 27.5895)
  line L1558 (5.1034, 27.5895) -> (5.0812, 27.6382)
  line L1559 (5.0812, 27.6382) -> (5.0787, 27.6559)
  line L1560 (5.0787, 27.6559) -> (5.0724, 27.6728)
  line L1561 (5.0724, 27.6728) -> (5.0686, 27.7261)
  line L1562 (5.0686, 27.7261) -> (5.061, 27.779)
  line L1563 (5.061, 27.779) -> (5.061, 28.5741)
  line L1564 (5.061, 28.5741) -> (4.711, 28.5741)
  line L1565 (4.711, 28.5741) -> (4.711, 30.2741)
  line L1566 (4.711, 30.2741) -> (6.411, 30.2741)
  line L1567 (6.411, 30.2741) -> (6.411, 28.5741)
  line L1568 (6.7817, 23.084) -> (6.9508, 23.0249)
  line L1569 (6.9508, 23.0249) -> (7.1025, 22.9296)
  line L1570 (7.1025, 22.9296) -> (7.2291, 22.8029)
  line L1571 (7.2291, 22.8029) -> (7.3244, 22.6512)
  line L1572 (7.3244, 22.6512) -> (7.3836, 22.4821)
  line L1573 (7.3836, 22.4821) -> (7.4037, 22.3041)
  line L1574 (7.4037, 22.3041) -> (7.3836, 22.1261)
  line L1575 (7.3836, 22.1261) -> (7.3244, 21.957)
  line L1576 (7.3244, 21.957) -> (7.2291, 21.8053)
  line L1577 (7.2291, 21.8053) -> (7.1025, 21.6786)
  line L1578 (7.1025, 21.6786) -> (6.9508, 21.5833)
  line L1579 (6.9508, 21.5833) -> (6.7817, 21.5241)
  line L1580 (6.7817, 21.5241) -> (6.6037, 21.5041)
  line L1581 (6.6037, 21.5041) -> (6.4256, 21.5241)
  line L1582 (6.4256, 21.5241) -> (6.2566, 21.5833)
  line L1583 (6.2566, 21.5833) -> (6.1049, 21.6786)
  line L1584 (6.1049, 21.6786) -> (5.9782, 21.8053)
  line L1585 (5.9782, 21.8053) -> (5.8829, 21.957)
  line L1586 (5.8829, 21.957) -> (5.8237, 22.1261)
  line L1587 (5.8237, 22.1261) -> (5.8037, 22.3041)
  line L1588 (5.8037, 22.3041) -> (5.8237, 22.4821)
  line L1589 (5.8237, 22.4821) -> (5.8829, 22.6512)
  line L1590 (5.8829, 22.6512) -> (5.9782, 22.8029)
  line L1591 (5.9782, 22.8029) -> (6.1049, 22.9296)
  line L1592 (6.1049, 22.9296) -> (6.2566, 23.0249)
  line L1593 (6.2566, 23.0249) -> (6.4256, 23.084)
  line L1594 (6.4256, 23.084) -> (6.6037, 23.1041)
  line L1595 (6.6037, 23.1041) -> (6.7817, 23.084)
  line L1596 (4.0637, 23.1041) -> (4.2417, 23.084)
  line L1597 (4.2417, 23.084) -> (4.4108, 23.0249)
  line L1598 (4.4108, 23.0249) -> (4.5625, 22.9296)
  line L1599 (4.5625, 22.9296) -> (4.6891, 22.8029)
  line L1600 (4.6891, 22.8029) -> (4.7844, 22.6512)
  line L1601 (4.7844, 22.6512) -> (4.8436, 22.4821)
  line L1602 (4.8436, 22.4821) -> (4.8637, 22.3041)
  line L1603 (4.8637, 22.3041) -> (4.8436, 22.1261)
  line L1604 (4.8436, 22.1261) -> (4.7844, 21.957)
  line L1605 (4.7844, 21.957) -> (4.6891, 21.8053)
  line L1606 (4.6891, 21.8053) -> (4.5625, 21.6786)
  line L1607 (4.5625, 21.6786) -> (4.4108, 21.5833)
  line L1608 (4.4108, 21.5833) -> (4.2417, 21.5241)
  line L1609 (4.2417, 21.5241) -> (4.0637, 21.5041)
  line L1610 (4.0637, 21.5041) -> (3.8856, 21.5241)
  line L1611 (3.8856, 21.5241) -> (3.7166, 21.5833)
  line L1612 (3.7166, 21.5833) -> (3.5649, 21.6786)
  line L1613 (3.5649, 21.6786) -> (3.4382, 21.8053)
  line L1614 (3.4382, 21.8053) -> (3.3429, 21.957)
  line L1615 (3.3429, 21.957) -> (3.2837, 22.1261)
  line L1616 (3.2837, 22.1261) -> (3.2637, 22.3041)
  line L1617 (3.2637, 22.3041) -> (3.2837, 22.4821)
  line L1618 (3.2837, 22.4821) -> (3.3429, 22.6512)
  line L1619 (3.3429, 22.6512) -> (3.4382, 22.8029)
  line L1620 (3.4382, 22.8029) -> (3.5649, 22.9296)
  line L1621 (3.5649, 22.9296) -> (3.7166, 23.0249)
  line L1622 (3.7166, 23.0249) -> (3.8856, 23.084)
  line L1623 (3.8856, 23.084) -> (4.0637, 23.1041)
  line L1624 (55.32, 31.15) -> (54.3271, 31.15)
  line L1625 (54.3271, 31.15) -> (51.4236, 28.2464)
  line L1626 (51.4236, 28.2464) -> (51.3807, 28.2144)
  line L1627 (51.3807, 28.2144) -> (51.3403, 28.1794)
  line L1628 (51.3403, 28.1794) -> (51.324, 28.1719)
  line L1629 (51.324, 28.1719) -> (51.3096, 28.1612)
  line L1630 (51.3096, 28.1612) -> (51.2595, 28.1425)
  line L1631 (51.2595, 28.1425) -> (51.2109, 28.1203)
  line L1632 (51.2109, 28.1203) -> (51.1931, 28.1177)
  line L1633 (51.1931, 28.1177) -> (51.1763, 28.1114)
  line L1634 (51.1763, 28.1114) -> (51.1229, 28.1076)
  line L1635 (51.1229, 28.1076) -> (51.07, 28.1)
  line L1636 (51.07, 28.1) -> (29.1343, 28.1)
  line L1637 (29.1343, 28.1) -> (29.0088, 27.9745)
  line L1638 (29.0088, 27.9745) -> (28.8571, 27.8792)
  line L1639 (28.8571, 27.8792) -> (28.688, 27.8201)
  line L1640 (28.688, 27.8201) -> (28.51, 27.8)
  line L1641 (28.51, 27.8) -> (28.332, 27.8201)
  line L1642 (28.332, 27.8201) -> (28.1629, 27.8792)
  line L1643 (28.1629, 27.8792) -> (28.0112, 27.9745)
  line L1644 (28.0112, 27.9745) -> (27.8845, 28.1012)
  line L1645 (27.8845, 28.1012) -> (27.7892, 28.2529)
  line L1646 (27.7892, 28.2529) -> (27.7301, 28.422)
  line L1647 (27.7301, 28.422) -> (27.71, 28.6)
  line L1648 (27.71, 28.6) -> (27.7301, 28.778)
  line L1649 (27.7301, 28.778) -> (27.7892, 28.9471)
  line L1650 (27.7892, 28.9471) -> (27.8845, 29.0988)
  line L1651 (27.8845, 29.0988) -> (28.0112, 29.2255)
  line L1652 (28.0112, 29.2255) -> (28.1629, 29.3208)
  line L1653 (28.1629, 29.3208) -> (28.332, 29.3799)
  line L1654 (28.332, 29.3799) -> (28.51, 29.4)
  line L1655 (28.51, 29.4) -> (28.688, 29.3799)
  line L1656 (28.688, 29.3799) -> (28.8571, 29.3208)
  line L1657 (28.8571, 29.3208) -> (29.0088, 29.2255)
  line L1658 (29.0088, 29.2255) -> (29.1343, 29.1)
  line L1659 (29.1343, 29.1) -> (50.8629, 29.1)
  line L1660 (50.8629, 29.1) -> (53.62, 31.8571)
  line L1661 (53.62, 31.8571) -> (53.62, 32.85)
  line L1662 (53.62, 32.85) -> (55.32, 32.85)
  line L1663 (55.32, 32.85) -> (55.32, 31.15)
  line L1664 (62.268, 32.7799) -> (62.4371, 32.7208)
  line L1665 (62.4371, 32.7208) -> (62.5888, 32.6255)
  line L1666 (62.5888, 32.6255) -> (62.7155, 32.4988)
  line L1667 (62.7155, 32.4988) -> (62.8108, 32.3471)
  line L1668 (62.8108, 32.3471) -> (62.8699, 32.178)
  line L1669 (62.8699, 32.178) -> (62.89, 32)
  line L1670 (62.89, 32) -> (62.8699, 31.822)
  line L1671 (62.8699, 31.822) -> (62.8108, 31.6529)
  line L1672 (62.8108, 31.6529) -> (62.7155, 31.5012)
  line L1673 (62.7155, 31.5012) -> (62.5888, 31.3745)
  line L1674 (62.5888, 31.3745) -> (62.4371, 31.2792)
  line L1675 (62.4371, 31.2792) -> (62.268, 31.2201)
  line L1676 (62.268, 31.2201) -> (62.09, 31.2)
  line L1677 (62.09, 31.2) -> (61.912, 31.2201)
  line L1678 (61.912, 31.2201) -> (61.7429, 31.2792)
  line L1679 (61.7429, 31.2792) -> (61.5912, 31.3745)
  line L1680 (61.5912, 31.3745) -> (61.4645, 31.5012)
  line L1681 (61.4645, 31.5012) -> (61.3692, 31.6529)
  line L1682 (61.3692, 31.6529) -> (61.3101, 31.822)
  line L1683 (61.3101, 31.822) -> (61.29, 32)
  line L1684 (61.29, 32) -> (61.3101, 32.178)
  line L1685 (61.3101, 32.178) -> (61.3692, 32.3471)
  line L1686 (61.3692, 32.3471) -> (61.4645, 32.4988)
  line L1687 (61.4645, 32.4988) -> (61.5912, 32.6255)
  line L1688 (61.5912, 32.6255) -> (61.7429, 32.7208)
  line L1689 (61.7429, 32.7208) -> (61.912, 32.7799)
  line L1690 (61.912, 32.7799) -> (62.09, 32.8)
  line L1691 (62.09, 32.8) -> (62.268, 32.7799)
  line L1692 (59.728, 32.7799) -> (59.8971, 32.7208)
  line L1693 (59.8971, 32.7208) -> (60.0488, 32.6255)
  line L1694 (60.0488, 32.6255) -> (60.1755, 32.4988)
  line L1695 (60.1755, 32.4988) -> (60.2708, 32.3471)
  line L1696 (60.2708, 32.3471) -> (60.3299, 32.178)
  line L1697 (60.3299, 32.178) -> (60.35, 32)
  line L1698 (60.35, 32) -> (60.3299, 31.822)
  line L1699 (60.3299, 31.822) -> (60.2708, 31.6529)
  line L1700 (60.2708, 31.6529) -> (60.1755, 31.5012)
  line L1701 (60.1755, 31.5012) -> (60.0488, 31.3745)
  line L1702 (60.0488, 31.3745) -> (59.8971, 31.2792)
  line L1703 (59.8971, 31.2792) -> (59.728, 31.2201)
  line L1704 (59.728, 31.2201) -> (59.55, 31.2)
  line L1705 (59.55, 31.2) -> (59.372, 31.2201)
  line L1706 (59.372, 31.2201) -> (59.2029, 31.2792)
  line L1707 (59.2029, 31.2792) -> (59.0512, 31.3745)
  line L1708 (59.0512, 31.3745) -> (58.9245, 31.5012)
  line L1709 (58.9245, 31.5012) -> (58.8292, 31.6529)
  line L1710 (58.8292, 31.6529) -> (58.7701, 31.822)
  line L1711 (58.7701, 31.822) -> (58.75, 32)
  line L1712 (58.75, 32) -> (58.7701, 32.178)
  line L1713 (58.7701, 32.178) -> (58.8292, 32.3471)
  line L1714 (58.8292, 32.3471) -> (58.9245, 32.4988)
  line L1715 (58.9245, 32.4988) -> (59.0512, 32.6255)
  line L1716 (59.0512, 32.6255) -> (59.2029, 32.7208)
  line L1717 (59.2029, 32.7208) -> (59.372, 32.7799)
  line L1718 (59.372, 32.7799) -> (59.55, 32.8)
  line L1719 (59.55, 32.8) -> (59.728, 32.7799)
  line L1720 (42.2425, 34.5309) -> (42.479, 34.4741)
  line L1721 (42.479, 34.4741) -> (42.7037, 34.3811)
  line L1722 (42.7037, 34.3811) -> (42.9111, 34.254)
  line L1723 (42.9111, 34.254) -> (43.096, 34.096)
  line L1724 (43.096, 34.096) -> (43.254, 33.9111)
  line L1725 (43.254, 33.9111) -> (43.3811, 33.7037)
  line L1726 (43.3811, 33.7037) -> (43.4741, 33.479)
  line L1727 (43.4741, 33.479) -> (43.5309, 33.2425)
  line L1728 (43.5309, 33.2425) -> (43.55, 33)
  line L1729 (43.55, 33) -> (43.5309, 32.7575)
  line L1730 (43.5309, 32.7575) -> (43.4741, 32.521)
  line L1731 (43.4741, 32.521) -> (43.3811, 32.2963)
  line L1732 (43.3811, 32.2963) -> (43.254, 32.0889)
  line L1733 (43.254, 32.0889) -> (43.096, 31.904)
  line L1734 (43.096, 31.904) -> (42.9111, 31.746)
  line L1735 (42.9111, 31.746) -> (42.7037, 31.6189)
  line L1736 (42.7037, 31.6189) -> (42.479, 31.5259)
  line L1737 (42.479, 31.5259) -> (42.2425, 31.4691)
  line L1738 (42.2425, 31.4691) -> (42, 31.45)
  line L1739 (42, 31.45) -> (41.7575, 31.4691)
  line L1740 (41.7575, 31.4691) -> (41.521, 31.5259)
  line L1741 (41.521, 31.5259) -> (41.2963, 31.6189)
  line L1742 (41.2963, 31.6189) -> (41.0889, 31.746)
  line L1743 (41.0889, 31.746) -> (40.904, 31.904)
  line L1744 (40.904, 31.904) -> (40.746, 32.0889)
  line L1745 (40.746, 32.0889) -> (40.6189, 32.2963)
  line L1746 (40.6189, 32.2963) -> (40.5259, 32.521)
  line L1747 (40.5259, 32.521) -> (40.4691, 32.7575)
  line L1748 (40.4691, 32.7575) -> (40.45, 33)
  line L1749 (40.45, 33) -> (40.4691, 33.2425)
  line L1750 (40.4691, 33.2425) -> (40.5259, 33.479)
  line L1751 (40.5259, 33.479) -> (40.6189, 33.7037)
  line L1752 (40.6189, 33.7037) -> (40.746, 33.9111)
  line L1753 (40.746, 33.9111) -> (40.904, 34.096)
  line L1754 (40.904, 34.096) -> (41.0889, 34.254)
  line L1755 (41.0889, 34.254) -> (41.2963, 34.3811)
  line L1756 (41.2963, 34.3811) -> (41.521, 34.4741)
  line L1757 (41.521, 34.4741) -> (41.7575, 34.5309)
  line L1758 (41.7575, 34.5309) -> (42, 34.55)
  line L1759 (42, 34.55) -> (42.2425, 34.5309)
  circle A0 centre (62.09, 32) radius 0.55
  circle A1 centre (59.55, 32) radius 0.55
  circle A2 centre (57.01, 32) radius 0.55
  circle A3 centre (54.47, 32) radius 0.55
  circle A4 centre (43.05, 18.71) radius 0.55
  circle A5 centre (43.05, 16.17) radius 0.55
  circle A6 centre (43.05, 13.63) radius 0.55
  circle A7 centre (43.05, 11.09) radius 0.55
  circle A8 centre (43.05, 8.55) radius 0.55
  circle A9 centre (43.05, 6.01) radius 0.55
  circle A10 centre (28.51, 28.6) radius 0.55
  circle A11 centre (20.89, 28.6) radius 0.55
  circle A12 centre (78.85, 18.9) radius 0.625
  circle A13 centre (78.85, 12.45) radius 0.625
  circle A14 centre (47.85, 12.45) radius 0.625
  circle A15 centre (47.85, 18.95) radius 0.625
  circle A16 centre (21.4306, 25.8601) radius 0.55
  circle A17 centre (29.0306, 25.8601) radius 0.55
  circle A18 centre (14.76, 26.2) radius 0.55
  circle A19 centre (7.14, 26.2) radius 0.55
  circle A20 centre (39.6237, 22.3041) radius 0.55
  circle A21 centre (37.0837, 22.3041) radius 0.55
  circle A22 centre (34.5437, 22.3041) radius 0.55
  circle A23 centre (32.0037, 22.3041) radius 0.55
  circle A24 centre (29.4637, 22.3041) radius 0.55
  circle A25 centre (26.9237, 22.3041) radius 0.55
  circle A26 centre (24.3837, 22.3041) radius 0.55
  circle A27 centre (21.8437, 22.3041) radius 0.55
  circle A28 centre (19.3037, 22.3041) radius 0.55
  circle A29 centre (16.7637, 22.3041) radius 0.55
  circle A30 centre (14.2237, 22.3041) radius 0.55
  circle A31 centre (11.6837, 22.3041) radius 0.55
  circle A32 centre (9.1437, 22.3041) radius 0.55
  circle A33 centre (6.6037, 22.3041) radius 0.55
  circle A34 centre (4.0637, 22.3041) radius 0.55
  circle A35 centre (4.0637, 7.0641) radius 0.55
  circle A36 centre (6.6037, 7.0641) radius 0.55
  circle A37 centre (9.1437, 7.0641) radius 0.55
  circle A38 centre (11.6837, 7.0641) radius 0.55
  circle A39 centre (14.2237, 7.0641) radius 0.55
  circle A40 centre (16.7637, 7.0641) radius 0.55
  circle A41 centre (19.3037, 7.0641) radius 0.55
  circle A42 centre (21.8437, 7.0641) radius 0.55
  circle A43 centre (24.3837, 7.0641) radius 0.55
  circle A44 centre (26.9237, 7.0641) radius 0.55
  circle A45 centre (29.4637, 7.0641) radius 0.55
  circle A46 centre (32.0037, 7.0641) radius 0.55
  circle A47 centre (34.5437, 7.0641) radius 0.55
  circle A48 centre (37.0837, 7.0641) radius 0.55
  circle A49 centre (39.6237, 7.0641) radius 0.55
  circle A50 centre (49.41, 4.7) radius 0.75
  circle A51 centre (69.9, 4.7) radius 0.75
  circle A52 centre (5.561, 29.4241) radius 0.55
  circle A53 centre (8.101, 29.4241) radius 0.55
  circle A54 centre (10.641, 29.4241) radius 0.55
  circle A55 centre (21.51, 31.95) radius 0.55
  circle A56 centre (13.89, 31.95) radius 0.55
  circle A57 centre (42, 33) radius 1.5
  circle A58 centre (80.5, 3.5) radius 1.5
  circle A59 centre (3.5, 3.5) radius 1.5
  line L1760 (0.127, 34.873) -> (83.873, 34.873)
  line L1761 (83.873, 34.873) -> (83.873, 0.127)
  line L1762 (83.873, 0.127) -> (0.127, 0.127)
  line L1763 (0.127, 0.127) -> (0.127, 34.873)
  line L1764 (61.9408, 25.0096) -> (63.9466, 28.484)
  line L1765 (63.9466, 28.484) -> (66.4472, 27.0403)
  line L1766 (66.4472, 27.0403) -> (64.4413, 23.5659)
  line L1767 (64.4413, 23.5659) -> (61.9408, 25.0096)
  line L1768 (59.2167, 28.484) -> (62.2531, 26.7309)
  line L1769 (62.2531, 26.7309) -> (60.9927, 24.5479)
  line L1770 (65.127, 28.484) -> (67.2534, 27.2563)
  line L1771 (67.2534, 27.2563) -> (65.8316, 24.7936)
  line L1772 (65.8316, 24.7936) -> (67.958, 23.5659)
  line L1773 (66.6378, 25.0096) -> (68.6437, 28.484)
  line L1774 (68.6437, 28.484) -> (69.9252, 27.7441)
  line L1775 (69.9252, 27.7441) -> (71.2068, 28.484)
  line L1776 (71.2068, 28.484) -> (73.2127, 25.0096)
  line L1777 (68.5572, 27.1539) -> (68.5572, 23.5659)
  line L1778 (68.5572, 23.5659) -> (69.9252, 23.5659)
  line L1779 (71.2932, 27.1539) -> (71.2932, 23.5659)
  line L1780 (71.2932, 23.5659) -> (69.9252, 23.5659)
  line L1781 (74.7234, 28.484) -> (72.597, 27.2563)
  line L1782 (72.597, 27.2563) -> (74.0188, 24.7936)
  line L1783 (74.0188, 24.7936) -> (71.8924, 23.5659)
  line L1784 (77.9097, 25.0096) -> (75.4091, 23.5659)
  line L1785 (75.4091, 23.5659) -> (73.4032, 27.0403)
  line L1786 (73.4032, 27.0403) -> (75.9038, 28.484)
  line L1787 (76.5852, 28.484) -> (79.4247, 23.5659)
  line L1788 (79.4247, 23.5659) -> (81.9252, 25.0096)
  line L1789 (57.9252, 23.5659) -> (60.3776, 27.8137)
  line L1790 (59.7424, 26.7135) -> (61.5597, 23.5659)
  line L1791 (74.4061, 25.3031) -> (76.9067, 26.7468)
  point P0 (0, 0)
  point P1 (3.6827, 14.1841)
  constraints: 3584 end point, 60 centre point, 60 horizontal, 54 vertical, 2 parallel, 1 perpendicular, 5380 other